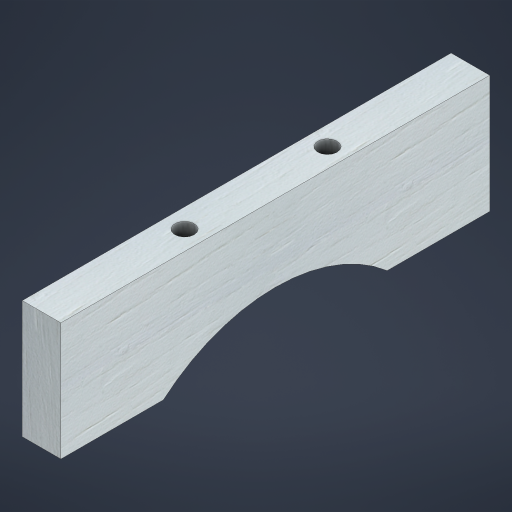
# Autodesk Inventor part: APM_003-1
Saved by Autodesk Inventor 2024 (Build 280153000, 153)
## iProperties
Created: 2023-02-14
Part Number: APM_003-1
Material: Genérico
Document SubType Name: Modeling
Designer: wob19
Density: 1 g/cm^3
Appearance: Valor por defecto
Author: wob19
Autodesk Inventor part; units mm, degrees
ref_plane "YZ Plane" through (0, 0, 0) normal (1, 0, 0) x (0, 1, 0)
ref_plane "XZ Plane" through (0, 0, 0) normal (0, 1, 0) x (-1, 0, 0)
ref_plane "XY Plane" through (0, 0, 0) normal (0, 0, 1) x (1, 0, 0)
sketch "Boceto1" plane through (0, 0, 0) normal (1, 0, 0) x (0, 1, 0)
  line L0 (27.5, -100) -> (-27.5, -100)
  line L1 (-27.5, -100) -> (-27.5, 100)
  line L2 (-27.5, 100) -> (27.5, 100)
  line L3 (27.5, 100) -> (27.5, -100)
  line L4 (27.5, -100) -> (-27.5, 100) construction
  line L5 (-27.5, -100) -> (27.5, 100) construction
  point P0 (0, 0)
  dimension "alto" = 55
  dimension "ancho" = 200
  constraints: 12 end point, 2 midpoint, 2 parallel, 1 horizontal, 1 perpendicular
  measures "alto" distance of L1.end L2.end
  measures "ancho" distance of L0.end L1.end
extrude "Extrusión1" add sketch "Boceto1" along normal blind 18
sketch "Boceto2" plane through (0, 27.5, 100) normal (0, 1, 0) x (1, 0, 0)
  circle A0 centre (9, 66.6667) radius 4.5
  circle A1 centre (9, 133.3333) radius 4.5
  line L0 (0, 0) -> (18, 0) projected
  line L1 (0, 200) -> (18, 200) projected
  line L2 (18, 200) -> (18, 0) projected
  point P0 (0, 100)
  dimension "d4" = 9
  dimension "d5" = 9
  dimension "alto1" = 66.6667
  dimension "d7" = 66.6667
  dimension "d8" = 9
  dimension "d9" = 9
  constraints: 2 centre point
  measures "d4" diameter of A0
  measures "d5" diameter of A1
  measures "alto1" distance from line of L0 A0.centre
  measures "d7" distance from line of L1 A1.centre
  measures "d8" distance from line of L2 A1.centre
  measures "d9" distance from line of L2 A0.centre
extrude "Extrusión2" cut sketch "Boceto2" against normal blind 6
sketch "Boceto3" plane through (18, 0, 0) normal (1, 0, 0) x (0, 0, -1)
  circle A0 centre (0, -88.1077) radius 80
  line L0 (-100, 27.5) -> (-100, -27.5) projected
  point P0 (0, 0)
  dimension "radio" = 160
  dimension "d14" = 100
  constraints: 1 centre point
  measures "radio" diameter of A0
  measures "d14" distance from line of A0.centre L0
extrude "Extrusión3" cut sketch "Boceto3" against normal blind 18
equation "\"d4\" = 0.5 * grosor"
equation "\"d5\" = d4"
equation "\"d7\" = alto1"
equation "\"d8\" = d9"
equation "\"d9\" = 0.5 * grosor"
equation "\"d10\" = 0.333333 * grosor"
equation "\"d14\" = 0.5 * ancho"
equation "\"d15\" = grosor"
equation "\"grosor\" = 18"
